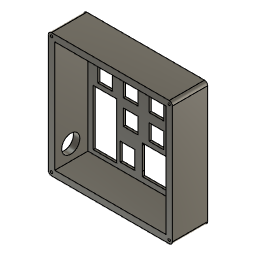
macro keyboard course ver 2 v2 (Autodesk Fusion 360 design; units mm, degrees)
Autodesk Fusion 360 part; units mm, degrees
note: some values were not read from the file. Set by a fixed rule: which sketch regions a step uses.
sketch "MacroKeyboard" plane through (0, 0, 0) normal (0, 1, 0) x (1, 0, 0)
  line L0 (24.38, -2.5067) -> (24.3899, -2.2367)
  line L1 (48.8951, -28.1499) -> (48.8951, -6.1499)
  line L2 (48.8951, -6.1499) -> (48.8951, -4.8499)
  line L3 (50.8951, -2.8499) -> (74.1951, -2.8499)
  line L4 (76.1951, -4.8499) -> (76.1951, -28.1499)
  line L5 (48.8951, -26.0859) -> (75.8951, -26.0859)
  line L6 (75.8951, -26.0859) -> (76.1951, -26.0859)
  line L7 (48.8951, -7.0859) -> (76.1951, -7.0859)
  line L8 (50.9271, -30.1499) -> (53.9271, -30.1499)
  line L9 (71.2271, -30.1499) -> (74.2271, -30.1499)
  line L10 (55.9271, -28.1499) -> (69.2271, -28.1499)
  line L11 (53.9271, -30.1499) -> (55.9271, -28.1499)
  line L12 (69.2271, -28.1499) -> (71.2271, -30.1499)
  line L13 (36.27, -14.02) -> (33.73, -14.02)
  line L14 (28.7501, -19.4501) -> (28.7501, -14.9001)
  line L15 (41.2502, -19.4501) -> (41.2502, -14.9001)
  line L16 (28.7501, -10.6) -> (28.7501, -6.05)
  line L17 (41.2502, -10.6) -> (41.2502, -6.05)
  line L18 (38.7003, -6.05) -> (41.2504, -6.05)
  line L19 (38.4002, -19.4501) -> (41.2501, -19.4501)
  line L20 (35.92, -19.4501) -> (36.62, -19.4501)
  line L21 (33.4, -19.4501) -> (34.1, -19.4501)
  line L22 (28.7501, -19.4501) -> (31.6, -19.4501)
  line L23 (33.725, -6.05) -> (36.275, -6.05)
  line L24 (28.7501, -6.05) -> (31.3, -6.05)
  line L25 (91.27, -14.02) -> (88.73, -14.02)
  line L26 (83.7501, -19.4501) -> (83.7501, -14.9001)
  line L27 (96.2502, -19.4501) -> (96.2502, -14.9001)
  line L28 (83.7501, -10.6) -> (83.7501, -6.05)
  line L29 (96.2502, -10.6) -> (96.2502, -6.05)
  line L30 (93.7003, -6.05) -> (96.2504, -6.05)
  line L31 (93.4002, -19.4501) -> (96.2501, -19.4501)
  line L32 (90.92, -19.4501) -> (91.62, -19.4501)
  line L33 (88.4, -19.4501) -> (89.1, -19.4501)
  line L34 (83.7501, -19.4501) -> (86.6, -19.4501)
  line L35 (88.725, -6.05) -> (91.275, -6.05)
  line L36 (83.7501, -6.05) -> (86.3, -6.05)
  arc A0 (48.8951, -28.1499) -> (50.8951, -30.1499) centre (50.8951, -28.1499) ccw
  arc A1 (50.8915, -2.8524) -> (48.8926, -4.8514) centre (50.8915, -4.8514) ccw
  arc A2 (76.2103, -4.8412) -> (74.2113, -2.8423) centre (74.2113, -4.8412) ccw
  arc A3 (74.1961, -30.1524) -> (76.1951, -28.1534) centre (74.1961, -28.1534) ccw
  arc A4 (36.27, -14.02) -> (33.73, -14.02) centre (35, -12.75) ccw
  arc A5 (91.27, -14.02) -> (88.73, -14.02) centre (90, -12.75) ccw
  circle A6 centre (35, -12.7501) radius 3
  circle A7 centre (90, -12.7501) radius 3
  circle A8 centre (34.1631, -39.5479) radius 0.7493
  circle A9 centre (34.1631, -39.5479) radius 1.1557
  circle A10 centre (40.5131, -37.0079) radius 0.7493
  circle A11 centre (40.5131, -37.0079) radius 1.1557
  circle A12 centre (58.2931, -39.5479) radius 0.7493
  circle A13 centre (58.2931, -39.5479) radius 1.1557
  circle A14 centre (64.6431, -37.0079) radius 0.7493
  circle A15 centre (64.6431, -37.0079) radius 1.1557
  circle A16 centre (82.4232, -39.5479) radius 0.7493
  circle A17 centre (82.4232, -39.5479) radius 1.1557
  circle A18 centre (88.7732, -37.0079) radius 0.7493
  circle A19 centre (88.7732, -37.0079) radius 1.1557
  circle A20 centre (10.287, -62.8524) radius 0.7493
  circle A21 centre (10.287, -62.8524) radius 1.1557
  circle A22 centre (16.637, -60.3124) radius 0.7493
  circle A23 centre (16.637, -60.3124) radius 1.1557
  circle A24 centre (34.163, -62.8524) radius 0.7493
  circle A25 centre (34.1631, -62.8524) radius 1.1557
  circle A26 centre (40.513, -60.3124) radius 0.7493
  circle A27 centre (40.5131, -60.3124) radius 1.1557
  circle A28 centre (58.2932, -62.8524) radius 0.7493
  circle A29 centre (58.2931, -62.8524) radius 1.1557
  circle A30 centre (64.6432, -60.3124) radius 0.7493
  circle A31 centre (64.6431, -60.3124) radius 1.1557
  circle A32 centre (82.4232, -62.8524) radius 0.7493
  circle A33 centre (82.4232, -62.8524) radius 1.1557
  circle A34 centre (88.7732, -60.3124) radius 0.7493
  circle A35 centre (88.7732, -60.3124) radius 1.1557
  circle A36 centre (10.287, -86.157) radius 0.7493
  circle A37 centre (10.287, -86.157) radius 1.1557
  circle A38 centre (16.637, -83.617) radius 0.7493
  circle A39 centre (16.637, -83.617) radius 1.1557
  circle A40 centre (34.1631, -86.157) radius 0.7493
  circle A41 centre (34.1631, -86.157) radius 1.1557
  circle A42 centre (40.5131, -83.617) radius 0.7493
  circle A43 centre (40.5131, -83.617) radius 1.1557
  circle A44 centre (58.2931, -86.157) radius 0.7493
  circle A45 centre (58.2931, -86.157) radius 1.1557
  circle A46 centre (64.6431, -83.617) radius 0.7493
  circle A47 centre (64.6431, -83.617) radius 1.1557
  circle A48 centre (82.4232, -86.157) radius 0.7493
  circle A49 centre (82.4232, -86.157) radius 1.1557
  circle A50 centre (88.7732, -83.617) radius 0.7493
  circle A51 centre (88.7732, -83.617) radius 1.1557
  arc A52 (5.0001, -4.1567) -> (5.0001, -3.0569) centre (5.0001, -3.6068) ccw
  arc A53 (4.9999, -3.0569) -> (4.9999, -4.1567) centre (4.9999, -3.6068) ccw
  line L37 (5.0001, -4.1567) -> (4.9999, -4.1567)
  line L38 (4.9999, -4.1567) -> (5.0001, -4.1567)
  line L39 (5.0001, -3.0569) -> (4.9999, -3.0569)
  line L40 (4.9999, -3.0569) -> (5.0001, -3.0569)
  arc A54 (5.0001, -6.6967) -> (5.0001, -5.5969) centre (5.0001, -6.1468) ccw
  arc A55 (4.9999, -5.5969) -> (4.9999, -6.6967) centre (4.9999, -6.1468) ccw
  line L41 (4.9999, -6.6967) -> (5.0001, -6.6967)
  line L42 (5.0001, -6.6967) -> (4.9999, -6.6967)
  line L43 (5.0001, -5.5969) -> (4.9999, -5.5969)
  line L44 (4.9999, -5.5969) -> (5.0001, -5.5969)
  arc A56 (5.0001, -9.2367) -> (5.0001, -8.1369) centre (5.0001, -8.6868) ccw
  arc A57 (4.9999, -8.1369) -> (4.9999, -9.2367) centre (4.9999, -8.6868) ccw
  line L45 (5.0001, -9.2367) -> (4.9999, -9.2367)
  line L46 (4.9999, -9.2367) -> (5.0001, -9.2367)
  line L47 (4.9999, -8.1369) -> (5.0001, -8.1369)
  line L48 (5.0001, -8.1369) -> (4.9999, -8.1369)
  arc A58 (5.0001, -11.7767) -> (5.0001, -10.6769) centre (5.0001, -11.2268) ccw
  arc A59 (4.9999, -10.6769) -> (4.9999, -11.7767) centre (4.9999, -11.2268) ccw
  line L49 (5.0001, -11.7767) -> (4.9999, -11.7767)
  line L50 (4.9999, -11.7767) -> (5.0001, -11.7767)
  line L51 (4.9999, -10.6769) -> (5.0001, -10.6769)
  line L52 (5.0001, -10.6769) -> (4.9999, -10.6769)
  arc A60 (5.0001, -14.3167) -> (5.0001, -13.2169) centre (5.0001, -13.7668) ccw
  arc A61 (4.9999, -13.2169) -> (4.9999, -14.3167) centre (4.9999, -13.7668) ccw
  line L53 (5.0001, -14.3167) -> (4.9999, -14.3167)
  line L54 (4.9999, -14.3167) -> (5.0001, -14.3167)
  line L55 (5.0001, -13.2169) -> (4.9999, -13.2169)
  line L56 (4.9999, -13.2169) -> (5.0001, -13.2169)
  arc A62 (5.0001, -16.8567) -> (5.0001, -15.7569) centre (5.0001, -16.3068) ccw
  arc A63 (4.9999, -15.7569) -> (4.9999, -16.8567) centre (4.9999, -16.3068) ccw
  line L57 (4.9999, -16.8567) -> (5.0001, -16.8567)
  line L58 (5.0001, -16.8567) -> (4.9999, -16.8567)
  line L59 (5.0001, -15.7569) -> (4.9999, -15.7569)
  line L60 (4.9999, -15.7569) -> (5.0001, -15.7569)
  arc A64 (5.0001, -19.3967) -> (5.0001, -18.2969) centre (5.0001, -18.8468) ccw
  arc A65 (4.9999, -18.2969) -> (4.9999, -19.3967) centre (4.9999, -18.8468) ccw
  line L61 (5.0001, -19.3967) -> (4.9999, -19.3967)
  line L62 (4.9999, -19.3967) -> (5.0001, -19.3967)
  line L63 (5.0001, -18.2969) -> (4.9999, -18.2969)
  line L64 (4.9999, -18.2969) -> (5.0001, -18.2969)
  arc A66 (5.0001, -21.9368) -> (5.0001, -20.8369) centre (5.0001, -21.3868) ccw
  arc A67 (4.9999, -20.8369) -> (4.9999, -21.9368) centre (4.9999, -21.3868) ccw
  line L65 (5.0001, -21.9368) -> (4.9999, -21.9368)
  line L66 (4.9999, -21.9368) -> (5.0001, -21.9368)
  line L67 (5.0001, -20.8369) -> (4.9999, -20.8369)
  line L68 (4.9999, -20.8369) -> (5.0001, -20.8369)
  arc A68 (5.0001, -24.4768) -> (5.0001, -23.3769) centre (5.0001, -23.9268) ccw
  arc A69 (4.9999, -23.3769) -> (4.9999, -24.4768) centre (4.9999, -23.9268) ccw
  line L69 (5.0001, -24.4768) -> (4.9999, -24.4768)
  line L70 (4.9999, -24.4768) -> (5.0001, -24.4768)
  line L71 (5.0001, -23.3769) -> (4.9999, -23.3769)
  line L72 (4.9999, -23.3769) -> (5.0001, -23.3769)
  arc A70 (5.0001, -27.0168) -> (5.0001, -25.9169) centre (5.0001, -26.4669) ccw
  arc A71 (4.9999, -25.9169) -> (4.9999, -27.0168) centre (4.9999, -26.4669) ccw
  line L73 (4.9999, -27.0168) -> (5.0001, -27.0168)
  line L74 (5.0001, -27.0168) -> (4.9999, -27.0168)
  line L75 (4.9999, -25.9169) -> (5.0001, -25.9169)
  line L76 (5.0001, -25.9169) -> (4.9999, -25.9169)
  arc A72 (5.0001, -29.5568) -> (5.0001, -28.4569) centre (5.0001, -29.0069) ccw
  arc A73 (4.9999, -28.4569) -> (4.9999, -29.5568) centre (4.9999, -29.0069) ccw
  line L77 (5.0001, -29.5568) -> (4.9999, -29.5568)
  line L78 (4.9999, -29.5568) -> (5.0001, -29.5568)
  line L79 (4.9999, -28.4569) -> (5.0001, -28.4569)
  line L80 (5.0001, -28.4569) -> (4.9999, -28.4569)
  arc A74 (5.0001, -32.0968) -> (5.0001, -30.997) centre (5.0001, -31.5469) ccw
  arc A75 (4.9999, -30.997) -> (4.9999, -32.0968) centre (4.9999, -31.5469) ccw
  line L81 (4.9999, -32.0968) -> (5.0001, -32.0968)
  line L82 (5.0001, -32.0968) -> (4.9999, -32.0968)
  line L83 (4.9999, -30.997) -> (5.0001, -30.997)
  line L84 (5.0001, -30.997) -> (4.9999, -30.997)
  arc A76 (5.0001, -34.6368) -> (5.0001, -33.537) centre (5.0001, -34.0869) ccw
  arc A77 (4.9999, -33.537) -> (4.9999, -34.6368) centre (4.9999, -34.0869) ccw
  line L85 (5.0001, -34.6368) -> (4.9999, -34.6368)
  line L86 (4.9999, -34.6368) -> (5.0001, -34.6368)
  line L87 (5.0001, -33.537) -> (4.9999, -33.537)
  line L88 (4.9999, -33.537) -> (5.0001, -33.537)
  arc A78 (5.0001, -37.1768) -> (5.0001, -36.077) centre (5.0001, -36.6269) ccw
  arc A79 (4.9999, -36.077) -> (4.9999, -37.1768) centre (4.9999, -36.6269) ccw
  line L89 (5.0001, -37.1768) -> (4.9999, -37.1768)
  line L90 (4.9999, -37.1768) -> (5.0001, -37.1768)
  line L91 (5.0001, -36.077) -> (4.9999, -36.077)
  line L92 (4.9999, -36.077) -> (5.0001, -36.077)
  arc A80 (5.0001, -39.7168) -> (5.0001, -38.617) centre (5.0001, -39.1669) ccw
  arc A81 (4.9999, -38.617) -> (4.9999, -39.7168) centre (4.9999, -39.1669) ccw
  line L93 (4.9999, -39.7168) -> (5.0001, -39.7168)
  line L94 (5.0001, -39.7168) -> (4.9999, -39.7168)
  line L95 (5.0001, -38.617) -> (4.9999, -38.617)
  line L96 (4.9999, -38.617) -> (5.0001, -38.617)
  arc A82 (5.0001, -42.2568) -> (5.0001, -41.157) centre (5.0001, -41.7069) ccw
  arc A83 (4.9999, -41.157) -> (4.9999, -42.2568) centre (4.9999, -41.7069) ccw
  line L97 (4.9999, -42.2568) -> (5.0001, -42.2568)
  line L98 (5.0001, -42.2568) -> (4.9999, -42.2568)
  line L99 (4.9999, -41.157) -> (5.0001, -41.157)
  line L100 (5.0001, -41.157) -> (4.9999, -41.157)
  arc A84 (5.0001, -44.7968) -> (5.0001, -43.697) centre (5.0001, -44.2469) ccw
  arc A85 (4.9999, -43.697) -> (4.9999, -44.7968) centre (4.9999, -44.2469) ccw
  line L101 (4.9999, -44.7968) -> (5.0001, -44.7968)
  line L102 (5.0001, -44.7968) -> (4.9999, -44.7968)
  line L103 (4.9999, -43.697) -> (5.0001, -43.697)
  line L104 (5.0001, -43.697) -> (4.9999, -43.697)
  arc A86 (5.0001, -47.3368) -> (5.0001, -46.237) centre (5.0001, -46.7869) ccw
  arc A87 (4.9999, -46.237) -> (4.9999, -47.3368) centre (4.9999, -46.7869) ccw
  line L105 (5.0001, -47.3368) -> (4.9999, -47.3368)
  line L106 (4.9999, -47.3368) -> (5.0001, -47.3368)
  line L107 (4.9999, -46.237) -> (5.0001, -46.237)
  line L108 (5.0001, -46.237) -> (4.9999, -46.237)
  arc A88 (5.0001, -49.8768) -> (5.0001, -48.777) centre (5.0001, -49.3269) ccw
  arc A89 (4.9999, -48.777) -> (4.9999, -49.8768) centre (4.9999, -49.3269) ccw
  line L109 (4.9999, -49.8768) -> (5.0001, -49.8768)
  line L110 (5.0001, -49.8768) -> (4.9999, -49.8768)
  line L111 (5.0001, -48.777) -> (4.9999, -48.777)
  line L112 (4.9999, -48.777) -> (5.0001, -48.777)
  arc A90 (5.0001, -52.4168) -> (5.0001, -51.317) centre (5.0001, -51.8669) ccw
  arc A91 (4.9999, -51.317) -> (4.9999, -52.4168) centre (4.9999, -51.8669) ccw
  line L113 (4.9999, -52.4168) -> (5.0001, -52.4168)
  line L114 (5.0001, -52.4168) -> (4.9999, -52.4168)
  line L115 (4.9999, -51.317) -> (5.0001, -51.317)
  line L116 (5.0001, -51.317) -> (4.9999, -51.317)
  arc A92 (22.7799, -51.317) -> (22.7799, -52.4168) centre (22.7799, -51.8669) ccw
  arc A93 (22.7802, -52.4168) -> (22.7802, -51.317) centre (22.7802, -51.8669) ccw
  line L117 (22.7799, -51.317) -> (22.7802, -51.317)
  line L118 (22.7802, -51.317) -> (22.7799, -51.317)
  line L119 (22.7799, -52.4168) -> (22.7802, -52.4168)
  line L120 (22.7802, -52.4168) -> (22.7799, -52.4168)
  arc A94 (22.7799, -48.777) -> (22.7799, -49.8768) centre (22.7799, -49.3269) ccw
  arc A95 (22.7802, -49.8768) -> (22.7802, -48.777) centre (22.7802, -49.3269) ccw
  line L121 (22.7799, -48.777) -> (22.7802, -48.777)
  line L122 (22.7802, -48.777) -> (22.7799, -48.777)
  line L123 (22.7799, -49.8768) -> (22.7802, -49.8768)
  line L124 (22.7802, -49.8768) -> (22.7799, -49.8768)
  arc A96 (22.7799, -46.237) -> (22.7799, -47.3368) centre (22.7799, -46.7869) ccw
  arc A97 (22.7802, -47.3368) -> (22.7802, -46.237) centre (22.7802, -46.7869) ccw
  line L125 (22.7802, -46.237) -> (22.7799, -46.237)
  line L126 (22.7799, -46.237) -> (22.7802, -46.237)
  line L127 (22.7802, -47.3368) -> (22.7799, -47.3368)
  line L128 (22.7799, -47.3368) -> (22.7802, -47.3368)
  arc A98 (22.7799, -43.697) -> (22.7799, -44.7968) centre (22.7799, -44.2469) ccw
  arc A99 (22.7802, -44.7968) -> (22.7802, -43.697) centre (22.7802, -44.2469) ccw
  line L129 (22.7802, -43.697) -> (22.7799, -43.697)
  line L130 (22.7799, -43.697) -> (22.7802, -43.697)
  line L131 (22.7799, -44.7968) -> (22.7802, -44.7968)
  line L132 (22.7802, -44.7968) -> (22.7799, -44.7968)
  arc A100 (22.7799, -41.157) -> (22.7799, -42.2568) centre (22.7799, -41.7069) ccw
  arc A101 (22.7802, -42.2568) -> (22.7802, -41.157) centre (22.7802, -41.7069) ccw
  line L133 (22.7799, -41.157) -> (22.7802, -41.157)
  line L134 (22.7802, -41.157) -> (22.7799, -41.157)
  line L135 (22.7802, -42.2568) -> (22.7799, -42.2568)
  line L136 (22.7799, -42.2568) -> (22.7802, -42.2568)
  arc A102 (22.7799, -38.617) -> (22.7799, -39.7168) centre (22.7799, -39.1669) ccw
  arc A103 (22.7802, -39.7168) -> (22.7802, -38.617) centre (22.7802, -39.1669) ccw
  line L137 (22.7799, -38.617) -> (22.7802, -38.617)
  line L138 (22.7802, -38.617) -> (22.7799, -38.617)
  line L139 (22.7802, -39.7168) -> (22.7799, -39.7168)
  line L140 (22.7799, -39.7168) -> (22.7802, -39.7168)
  arc A104 (22.7799, -36.077) -> (22.7799, -37.1768) centre (22.7799, -36.6269) ccw
  arc A105 (22.7802, -37.1768) -> (22.7802, -36.077) centre (22.7802, -36.6269) ccw
  line L141 (22.7802, -36.077) -> (22.7799, -36.077)
  line L142 (22.7799, -36.077) -> (22.7802, -36.077)
  line L143 (22.7802, -37.1768) -> (22.7799, -37.1768)
  line L144 (22.7799, -37.1768) -> (22.7802, -37.1768)
  arc A106 (22.7799, -33.537) -> (22.7799, -34.6368) centre (22.7799, -34.0869) ccw
  arc A107 (22.7802, -34.6368) -> (22.7802, -33.537) centre (22.7802, -34.0869) ccw
  line L145 (22.7799, -33.537) -> (22.7802, -33.537)
  line L146 (22.7802, -33.537) -> (22.7799, -33.537)
  line L147 (22.7802, -34.6368) -> (22.7799, -34.6368)
  line L148 (22.7799, -34.6368) -> (22.7802, -34.6368)
  arc A108 (22.7799, -30.997) -> (22.7799, -32.0968) centre (22.7799, -31.5469) ccw
  arc A109 (22.7802, -32.0968) -> (22.7802, -30.997) centre (22.7802, -31.5469) ccw
  line L149 (22.7802, -30.997) -> (22.7799, -30.997)
  line L150 (22.7799, -30.997) -> (22.7802, -30.997)
  line L151 (22.7802, -32.0968) -> (22.7799, -32.0968)
  line L152 (22.7799, -32.0968) -> (22.7802, -32.0968)
  arc A110 (22.7799, -28.4569) -> (22.7799, -29.5568) centre (22.7799, -29.0069) ccw
  arc A111 (22.7802, -29.5568) -> (22.7802, -28.4569) centre (22.7802, -29.0069) ccw
  line L153 (22.7802, -28.4569) -> (22.7799, -28.4569)
  line L154 (22.7799, -28.4569) -> (22.7802, -28.4569)
  line L155 (22.7799, -29.5568) -> (22.7802, -29.5568)
  line L156 (22.7802, -29.5568) -> (22.7799, -29.5568)
  arc A112 (22.7799, -25.9169) -> (22.7799, -27.0168) centre (22.7799, -26.4669) ccw
  arc A113 (22.7802, -27.0168) -> (22.7802, -25.9169) centre (22.7802, -26.4669) ccw
  line L157 (22.7802, -25.9169) -> (22.7799, -25.9169)
  line L158 (22.7799, -25.9169) -> (22.7802, -25.9169)
  line L159 (22.7799, -27.0168) -> (22.7802, -27.0168)
  line L160 (22.7802, -27.0168) -> (22.7799, -27.0168)
  arc A114 (22.7799, -23.3769) -> (22.7799, -24.4768) centre (22.7799, -23.9268) ccw
  arc A115 (22.7802, -24.4768) -> (22.7802, -23.3769) centre (22.7802, -23.9268) ccw
  line L161 (22.7799, -23.3769) -> (22.7802, -23.3769)
  line L162 (22.7802, -23.3769) -> (22.7799, -23.3769)
  line L163 (22.7799, -24.4768) -> (22.7802, -24.4768)
  line L164 (22.7802, -24.4768) -> (22.7799, -24.4768)
  arc A116 (22.7799, -20.8369) -> (22.7799, -21.9368) centre (22.7799, -21.3868) ccw
  arc A117 (22.7802, -21.9368) -> (22.7802, -20.8369) centre (22.7802, -21.3868) ccw
  line L165 (22.7802, -20.8369) -> (22.7799, -20.8369)
  line L166 (22.7799, -20.8369) -> (22.7802, -20.8369)
  line L167 (22.7799, -21.9368) -> (22.7802, -21.9368)
  line L168 (22.7802, -21.9368) -> (22.7799, -21.9368)
  arc A118 (22.7799, -18.2969) -> (22.7799, -19.3967) centre (22.7799, -18.8468) ccw
  arc A119 (22.7802, -19.3967) -> (22.7802, -18.2969) centre (22.7802, -18.8468) ccw
  line L169 (22.7799, -18.2969) -> (22.7802, -18.2969)
  line L170 (22.7802, -18.2969) -> (22.7799, -18.2969)
  line L171 (22.7802, -19.3967) -> (22.7799, -19.3967)
  line L172 (22.7799, -19.3967) -> (22.7802, -19.3967)
  arc A120 (22.7799, -15.7569) -> (22.7799, -16.8567) centre (22.7799, -16.3068) ccw
  arc A121 (22.7802, -16.8567) -> (22.7802, -15.7569) centre (22.7802, -16.3068) ccw
  line L173 (22.7799, -15.7569) -> (22.7802, -15.7569)
  line L174 (22.7802, -15.7569) -> (22.7799, -15.7569)
  line L175 (22.7802, -16.8567) -> (22.7799, -16.8567)
  line L176 (22.7799, -16.8567) -> (22.7802, -16.8567)
  arc A122 (22.7799, -13.2169) -> (22.7799, -14.3167) centre (22.7799, -13.7668) ccw
  arc A123 (22.7802, -14.3167) -> (22.7802, -13.2169) centre (22.7802, -13.7668) ccw
  line L177 (22.7802, -13.2169) -> (22.7799, -13.2169)
  line L178 (22.7799, -13.2169) -> (22.7802, -13.2169)
  line L179 (22.7802, -14.3167) -> (22.7799, -14.3167)
  line L180 (22.7799, -14.3167) -> (22.7802, -14.3167)
  arc A124 (22.7799, -10.6769) -> (22.7799, -11.7767) centre (22.7799, -11.2268) ccw
  arc A125 (22.7802, -11.7767) -> (22.7802, -10.6769) centre (22.7802, -11.2268) ccw
  line L181 (22.7802, -10.6769) -> (22.7799, -10.6769)
  line L182 (22.7799, -10.6769) -> (22.7802, -10.6769)
  line L183 (22.7799, -11.7767) -> (22.7802, -11.7767)
  line L184 (22.7802, -11.7767) -> (22.7799, -11.7767)
  arc A126 (22.7799, -8.1369) -> (22.7799, -9.2367) centre (22.7799, -8.6868) ccw
  arc A127 (22.7802, -9.2367) -> (22.7802, -8.1369) centre (22.7802, -8.6868) ccw
  line L185 (22.7799, -8.1369) -> (22.7802, -8.1369)
  line L186 (22.7802, -8.1369) -> (22.7799, -8.1369)
  line L187 (22.7799, -9.2367) -> (22.7802, -9.2367)
  line L188 (22.7802, -9.2367) -> (22.7799, -9.2367)
  arc A128 (22.7799, -5.5969) -> (22.7799, -6.6967) centre (22.7799, -6.1468) ccw
  arc A129 (22.7802, -6.6967) -> (22.7802, -5.5969) centre (22.7802, -6.1468) ccw
  line L189 (22.7799, -5.5969) -> (22.7802, -5.5969)
  line L190 (22.7802, -5.5969) -> (22.7799, -5.5969)
  line L191 (22.7802, -6.6967) -> (22.7799, -6.6967)
  line L192 (22.7799, -6.6967) -> (22.7802, -6.6967)
  arc A130 (22.7799, -3.0569) -> (22.7799, -4.1567) centre (22.7799, -3.6068) ccw
  arc A131 (22.7802, -4.1567) -> (22.7802, -3.0569) centre (22.7802, -3.6068) ccw
  line L193 (22.7802, -3.0569) -> (22.7799, -3.0569)
  line L194 (22.7799, -3.0569) -> (22.7802, -3.0569)
  line L195 (22.7802, -4.1567) -> (22.7799, -4.1567)
  line L196 (22.7799, -4.1567) -> (22.7802, -4.1567)
  arc A132 (11.8999, -51.6367) -> (10.8001, -51.6367) centre (11.35, -51.6367) ccw
  arc A133 (10.8001, -51.6369) -> (11.8999, -51.6369) centre (11.35, -51.6369) ccw
  line L197 (10.8001, -51.6369) -> (10.8001, -51.6367)
  line L198 (10.8001, -51.6367) -> (10.8001, -51.6369)
  line L199 (11.8999, -51.6367) -> (11.8999, -51.6369)
  line L200 (11.8999, -51.6369) -> (11.8999, -51.6367)
  arc A134 (14.4399, -51.6367) -> (13.3401, -51.6367) centre (13.89, -51.6367) ccw
  arc A135 (13.3401, -51.6369) -> (14.4399, -51.6369) centre (13.89, -51.6369) ccw
  line L201 (13.3401, -51.6369) -> (13.3401, -51.6367)
  line L202 (13.3401, -51.6367) -> (13.3401, -51.6369)
  line L203 (14.4399, -51.6367) -> (14.4399, -51.6369)
  line L204 (14.4399, -51.6369) -> (14.4399, -51.6367)
  arc A136 (16.9799, -51.6367) -> (15.8801, -51.6367) centre (16.43, -51.6367) ccw
  arc A137 (15.8801, -51.6369) -> (16.9799, -51.6369) centre (16.43, -51.6369) ccw
  line L205 (15.8801, -51.6367) -> (15.8801, -51.6369)
  line L206 (15.8801, -51.6369) -> (15.8801, -51.6367)
  line L207 (16.9799, -51.6367) -> (16.9799, -51.6369)
  line L208 (16.9799, -51.6369) -> (16.9799, -51.6367)
  circle A138 centre (58.8011, -4.5499) radius 0.4572
  circle A139 centre (61.3411, -4.5491) radius 0.4572
  circle A140 centre (61.3411, -4.5491) radius 0.762
  circle A141 centre (63.8811, -4.5491) radius 0.4572
  circle A142 centre (63.8811, -4.5491) radius 0.762
  circle A143 centre (66.4211, -4.5491) radius 0.4572
  circle A144 centre (66.4211, -4.5491) radius 0.762
  circle A145 centre (32.5001, -5.7501) radius 0.6
  circle A146 centre (32.5001, -5.7501) radius 0.9
  circle A147 centre (37.5001, -5.7501) radius 0.6
  circle A148 centre (37.5001, -5.7501) radius 0.9
  circle A149 centre (32.5001, -20.2499) radius 0.6
  circle A150 centre (32.5001, -20.2499) radius 0.9
  circle A151 centre (35, -20.2499) radius 0.6
  circle A152 centre (35, -20.2499) radius 0.9
  circle A153 centre (37.5001, -20.2499) radius 0.6
  circle A154 centre (37.5001, -20.2499) radius 0.9
  arc A155 (28.6, -12.0501) -> (30, -12.0501) centre (29.3, -12.0501) ccw
  arc A156 (30, -13.4501) -> (28.6, -13.4501) centre (29.3, -13.4501) ccw
  line L209 (28.6, -13.4501) -> (28.6, -12.0501)
  line L210 (28.6, -12.0501) -> (28.6, -13.4501)
  line L211 (30, -13.4501) -> (30, -12.0501)
  line L212 (30, -12.0501) -> (30, -13.4501)
  arc A157 (40, -12.0501) -> (41.4, -12.0501) centre (40.7, -12.0501) ccw
  arc A158 (41.4, -13.4501) -> (40, -13.4501) centre (40.7, -13.4501) ccw
  line L213 (40, -12.0501) -> (40, -13.4501)
  line L214 (40, -13.4501) -> (40, -12.0501)
  line L215 (41.4, -12.0501) -> (41.4, -13.4501)
  line L216 (41.4, -13.4501) -> (41.4, -12.0501)
  circle A159 centre (87.5001, -5.7501) radius 0.6
  circle A160 centre (87.5001, -5.7501) radius 0.9
  circle A161 centre (92.5001, -5.7501) radius 0.6
  circle A162 centre (92.5001, -5.7501) radius 0.9
  circle A163 centre (87.5001, -20.2499) radius 0.6
  circle A164 centre (87.5001, -20.2499) radius 0.9
  circle A165 centre (90, -20.2499) radius 0.6
  circle A166 centre (90, -20.2499) radius 0.9
  circle A167 centre (92.5001, -20.2499) radius 0.6
  circle A168 centre (92.5001, -20.2499) radius 0.9
  arc A169 (83.6, -12.0501) -> (85, -12.0501) centre (84.3, -12.0501) ccw
  arc A170 (85, -13.4501) -> (83.6, -13.4501) centre (84.3, -13.4501) ccw
  line L217 (83.6, -12.0501) -> (83.6, -13.4501)
  line L218 (83.6, -13.4501) -> (83.6, -12.0501)
  line L219 (85, -13.4501) -> (85, -12.0501)
  line L220 (85, -12.0501) -> (85, -13.4501)
  arc A171 (95, -12.0501) -> (96.4, -12.0501) centre (95.7, -12.0501) ccw
  arc A172 (96.4, -13.4501) -> (95, -13.4501) centre (95.7, -13.4501) ccw
  line L221 (95, -13.4501) -> (95, -12.0501)
  line L222 (95, -12.0501) -> (95, -13.4501)
  line L223 (96.4, -12.0501) -> (96.4, -13.4501)
  line L224 (96.4, -13.4501) -> (96.4, -12.0501)
  circle A173 centre (11.2355, -28.4567) radius 0.2
  circle A174 centre (8.2985, -33.2898) radius 0.2
  circle A175 centre (12.0828, -85.3744) radius 0.2
  circle A176 centre (90, -16.6876) radius 0.2
  circle A177 centre (43.7206, -68.8435) radius 0.2
  circle A178 centre (6.6589, -46.5507) radius 0.2
  circle A179 centre (65.2781, -49.0729) radius 0.2
  circle A180 centre (7.7234, -36.6269) radius 0.2
  circle A181 centre (37.9731, -42.0879) radius 1.9939
  circle A182 centre (62.1031, -42.0879) radius 1.9939
  circle A183 centre (86.2332, -42.0879) radius 1.9939
  circle A184 centre (14.097, -65.3924) radius 1.9939
  circle A185 centre (37.9731, -65.3924) radius 1.9939
  circle A186 centre (62.1031, -65.3924) radius 1.9939
  circle A187 centre (86.2332, -65.3924) radius 1.9939
  circle A188 centre (14.097, -88.697) radius 1.9939
  circle A189 centre (37.9731, -88.697) radius 1.9939
  circle A190 centre (62.1031, -88.697) radius 1.9939
  circle A191 centre (86.2332, -88.697) radius 1.9939
  circle A192 centre (52.1971, -28.1179) radius 1.016
  circle A193 centre (72.8981, -28.1179) radius 1.016
  circle A194 centre (52.1971, -4.9174) radius 1.016
  circle A195 centre (72.8981, -4.9174) radius 1.016
  line L225 (-2, -102) -> (-2, 2)
  line L226 (-2, 2) -> (102, 2)
  line L227 (102, 2) -> (102, -102)
  line L228 (102, -102) -> (-2, -102)
  line L229 (24.8899, -1.7367) -> (2.8899, -1.7367)
  line L230 (2.8899, -1.7367) -> (2.8899, -53.7367)
  line L231 (2.8899, -53.7367) -> (24.8899, -53.7367)
  line L232 (24.8899, -53.7367) -> (24.8899, -1.7367)
  line L233 (20.947, -96.197) -> (7.247, -96.197)
  line L234 (7.247, -96.197) -> (7.247, -81.197)
  line L235 (7.247, -81.197) -> (20.947, -81.197)
  line L236 (20.947, -81.197) -> (20.947, -96.197)
  line L237 (20.947, -96.197) -> (7.247, -81.197) construction
  line L238 (7.247, -96.197) -> (20.947, -81.197) construction
  line L239 (44.8231, -96.197) -> (31.1231, -96.197)
  line L240 (31.1231, -96.197) -> (31.1231, -81.197)
  line L241 (31.1231, -81.197) -> (44.8231, -81.197)
  line L242 (44.8231, -81.197) -> (44.8231, -96.197)
  line L243 (44.8231, -96.197) -> (31.1231, -81.197) construction
  line L244 (31.1231, -96.197) -> (44.8231, -81.197) construction
  line L245 (20.947, -72.8924) -> (7.247, -72.8924)
  line L246 (7.247, -72.8924) -> (7.247, -57.8924)
  line L247 (7.247, -57.8924) -> (20.947, -57.8924)
  line L248 (20.947, -57.8924) -> (20.947, -72.8924)
  line L249 (20.947, -72.8924) -> (7.247, -57.8924) construction
  line L250 (7.247, -72.8924) -> (20.947, -57.8924) construction
  line L251 (44.8231, -72.8924) -> (31.1231, -72.8924)
  line L252 (31.1231, -72.8924) -> (31.1231, -57.8924)
  line L253 (31.1231, -57.8924) -> (44.8231, -57.8924)
  line L254 (44.8231, -57.8924) -> (44.8231, -72.8924)
  line L255 (44.8231, -72.8924) -> (31.1231, -57.8924) construction
  line L256 (31.1231, -72.8924) -> (44.8231, -57.8924) construction
  line L257 (44.8231, -49.5879) -> (31.1231, -49.5879)
  line L258 (31.1231, -49.5879) -> (31.1231, -34.5879)
  line L259 (31.1231, -34.5879) -> (44.8231, -34.5879)
  line L260 (44.8231, -34.5879) -> (44.8231, -49.5879)
  line L261 (44.8231, -49.5879) -> (31.1231, -34.5879) construction
  line L262 (31.1231, -49.5879) -> (44.8231, -34.5879) construction
  line L263 (68.9531, -96.197) -> (55.2531, -96.197)
  line L264 (55.2531, -96.197) -> (55.2531, -81.197)
  line L265 (55.2531, -81.197) -> (68.9531, -81.197)
  line L266 (68.9531, -81.197) -> (68.9531, -96.197)
  line L267 (68.9531, -96.197) -> (55.2531, -81.197) construction
  line L268 (55.2531, -96.197) -> (68.9531, -81.197) construction
  line L269 (93.0832, -96.197) -> (79.3832, -96.197)
  line L270 (79.3832, -96.197) -> (79.3832, -81.197)
  line L271 (79.3832, -81.197) -> (93.0832, -81.197)
  line L272 (93.0832, -81.197) -> (93.0832, -96.197)
  line L273 (93.0832, -96.197) -> (79.3832, -81.197) construction
  line L274 (79.3832, -96.197) -> (93.0832, -81.197) construction
  line L275 (68.9531, -72.8924) -> (55.2531, -72.8924)
  line L276 (55.2531, -72.8924) -> (55.2531, -57.8924)
  line L277 (55.2531, -57.8924) -> (68.9531, -57.8924)
  line L278 (68.9531, -57.8924) -> (68.9531, -72.8924)
  line L279 (68.9531, -72.8924) -> (55.2531, -57.8924) construction
  line L280 (55.2531, -72.8924) -> (68.9531, -57.8924) construction
  line L281 (93.0832, -72.8924) -> (79.3832, -72.8924)
  line L282 (79.3832, -72.8924) -> (79.3832, -57.8924)
  line L283 (79.3832, -57.8924) -> (93.0832, -57.8924)
  line L284 (93.0832, -57.8924) -> (93.0832, -72.8924)
  line L285 (93.0832, -72.8924) -> (79.3832, -57.8924) construction
  line L286 (79.3832, -72.8924) -> (93.0832, -57.8924) construction
  line L287 (68.9531, -49.5879) -> (55.2531, -49.5879)
  line L288 (55.2531, -49.5879) -> (55.2531, -34.5879)
  line L289 (55.2531, -34.5879) -> (68.9531, -34.5879)
  line L290 (68.9531, -34.5879) -> (68.9531, -49.5879)
  line L291 (68.9531, -49.5879) -> (55.2531, -34.5879) construction
  line L292 (55.2531, -49.5879) -> (68.9531, -34.5879) construction
  line L293 (93.0832, -49.5879) -> (79.3832, -49.5879)
  line L294 (79.3832, -49.5879) -> (79.3832, -34.5879)
  line L295 (79.3832, -34.5879) -> (93.0832, -34.5879)
  line L296 (93.0832, -34.5879) -> (93.0832, -49.5879)
  line L297 (93.0832, -49.5879) -> (79.3832, -34.5879) construction
  line L298 (79.3832, -49.5879) -> (93.0832, -34.5879) construction
  line L299 (50.8951, -28.1499) -> (74.2113, -4.8412)
  line L300 (74.2113, -4.8412) -> (74.1961, -28.1534)
  line L301 (74.1961, -28.1534) -> (50.8915, -4.8514)
  line L302 (76.1953, -30.1524) -> (48.9111, -30.1524)
  line L303 (48.9111, -30.1524) -> (48.9111, -2.8387)
  line L304 (48.9111, -2.8387) -> (76.1953, -2.8387)
  line L305 (76.1953, -2.8387) -> (76.1953, -30.1524)
  line L306 (76.1953, -30.1524) -> (48.9111, -2.8387) construction
  line L307 (48.9111, -30.1524) -> (76.1953, -2.8387) construction
  line L308 (96.75, -21.2501) -> (83.25, -21.2501)
  line L309 (83.25, -21.2501) -> (83.25, -4.2501)
  line L310 (83.25, -4.2501) -> (96.75, -4.2501)
  line L311 (96.75, -4.2501) -> (96.75, -21.2501)
  line L312 (96.75, -21.2501) -> (83.25, -4.2501) construction
  line L313 (83.25, -21.2501) -> (96.75, -4.2501) construction
  line L314 (41.85, -21.2501) -> (28.15, -21.2501)
  line L315 (28.15, -21.2501) -> (28.15, -4.2501)
  line L316 (28.15, -4.2501) -> (41.85, -4.2501)
  line L317 (41.85, -4.2501) -> (41.85, -21.2501)
  line L318 (41.85, -21.2501) -> (28.15, -4.2501) construction
  line L319 (28.15, -21.2501) -> (41.85, -4.2501) construction
  line L320 (108, 5) -> (108, -105)
  line L321 (105, -108) -> (-5, -108)
  line L322 (-8, -105) -> (-8, 5)
  line L323 (-5, 8) -> (105, 8)
  line L324 (102, 2) -> (108, 8)
  line L325 (-8, 8) -> (-2, 2)
  line L326 (-8, -108) -> (-2, -102)
  line L327 (102, -102) -> (108, -108)
  circle A196 centre (105, -105) radius 1.1
  circle A197 centre (105, 5) radius 1.1
  circle A198 centre (-5, 5) radius 1.1
  circle A199 centre (-5, -105) radius 1.1
  arc A200 (-5, 8) -> (-8, 5) centre (-5, 5) ccw
  arc A201 (108, 5) -> (105, 8) centre (105, 5) ccw
  arc A202 (105, -108) -> (108, -105) centre (105, -105) ccw
  arc A203 (-8, -105) -> (-5, -108) centre (-5, -105) ccw
  point P0 (14.097, -88.697)
  point P1 (37.9731, -88.697)
  point P2 (14.097, -65.3924)
  point P3 (37.9731, -65.3924)
  point P4 (37.9731, -42.0879)
  point P5 (62.1031, -88.697)
  point P6 (86.2332, -88.697)
  point P7 (62.1031, -65.3924)
  point P8 (86.2332, -65.3924)
  point P9 (62.1031, -42.0879)
  point P10 (86.2332, -42.0879)
  point P11 (62.5532, -16.4956)
  point P12 (90, -12.7501)
  point P13 (35, -12.7501)
  dimension "d3" = 13.7
  dimension "d4" = 15
  dimension "d5" = 13.7
  dimension "d6" = 15
  dimension "d7" = 13.7
  dimension "d8" = 15
  dimension "d9" = 13.7
  dimension "d10" = 15
  dimension "d11" = 13.7
  dimension "d12" = 15
  dimension "d13" = 13.7
  dimension "d14" = 15
  dimension "d15" = 13.7
  dimension "d16" = 15
  dimension "d17" = 13.7
  dimension "d18" = 15
  dimension "d19" = 13.7
  dimension "d20" = 15
  dimension "d21" = 13.7
  dimension "d22" = 15
  dimension "d23" = 13.7
  dimension "d24" = 15
  dimension "d25" = 13.5
  dimension "d26" = 17
  dimension "d27" = 13.7
  dimension "d28" = 17
  dimension "d30" = 2.2
  dimension "d31" = 2.2
  dimension "d32" = 2.2
  dimension "d33" = 2.2
  dimension "d46" = 3
  dimension "d47" = 3
  dimension "d48" = 3
  dimension "d49" = 3
  constraint horizontal L233
  constraint perpendicular L233 L234
  constraint parallel L233 L235
  constraint parallel L234 L236
  constraint coincident L237 P0
  constraint coincident L238 P0
  constraint coincident P0 A188.centre
  constraint horizontal L239
  constraint perpendicular L239 L240
  constraint parallel L239 L241
  constraint parallel L240 L242
  constraint coincident L243 P1
  constraint coincident L244 P1
  constraint coincident P1 A189.centre
  constraint horizontal L245
  constraint perpendicular L245 L246
  constraint parallel L245 L247
  constraint parallel L246 L248
  constraint coincident L249 P2
  constraint coincident L250 P2
  constraint coincident P2 A184.centre
  constraint horizontal L251
  constraint perpendicular L251 L252
  constraint parallel L251 L253
  constraint parallel L252 L254
  constraint coincident L255 P3
  constraint coincident L256 P3
  constraint coincident P3 A185.centre
  constraint horizontal L257
  constraint perpendicular L257 L258
  constraint parallel L257 L259
  constraint parallel L258 L260
  constraint coincident L261 P4
  constraint coincident L262 P4
  constraint coincident P4 A181.centre
  constraint horizontal L263
  constraint perpendicular L263 L264
  constraint parallel L263 L265
  constraint parallel L264 L266
  constraint coincident L267 P5
  constraint coincident L268 P5
  constraint coincident P5 A190.centre
  constraint horizontal L269
  constraint perpendicular L269 L270
  constraint parallel L269 L271
  constraint parallel L270 L272
  constraint coincident L273 P6
  constraint coincident L274 P6
  constraint coincident P6 A191.centre
  constraint horizontal L275
  constraint perpendicular L275 L276
  constraint parallel L275 L277
  constraint parallel L276 L278
  constraint coincident L279 P7
  constraint coincident L280 P7
  constraint coincident P7 A186.centre
  constraint horizontal L281
  constraint perpendicular L281 L282
  constraint parallel L281 L283
  constraint parallel L282 L284
  constraint coincident L285 P8
  constraint coincident L286 P8
  constraint coincident P8 A187.centre
  constraint horizontal L287
  constraint perpendicular L287 L288
  constraint parallel L287 L289
  constraint parallel L288 L290
  constraint coincident L291 P9
  constraint coincident L292 P9
  constraint coincident P9 A182.centre
  constraint horizontal L293
  constraint perpendicular L293 L294
  constraint parallel L293 L295
  constraint parallel L294 L296
  constraint coincident L297 P10
  constraint coincident L298 P10
  constraint coincident P10 A183.centre
  constraint coincident A0.centre L299.start
  constraint coincident A2.centre L299.end
  constraint coincident A3.centre L300.end
  constraint coincident A1.centre L301.end
  constraint horizontal L302
  constraint perpendicular L302 L303
  constraint parallel L302 L304
  constraint parallel L303 L305
  constraint coincident L306 P11
  constraint coincident L307 P11
  constraint midpoint L299 P11
  constraint horizontal L308
  constraint perpendicular L308 L309
  constraint parallel L308 L310
  constraint parallel L309 L311
  constraint coincident L312 P12
  constraint coincident L313 P12
  constraint coincident P12 A7.centre
  constraint horizontal L314
  constraint perpendicular L314 L315
  constraint parallel L314 L316
  constraint parallel L315 L317
  constraint coincident L318 P13
  constraint coincident L319 P13
  constraint coincident P13 A6.centre
  constraint perpendicular L324 L325
  constraint perpendicular L325 L326
  constraint midpoint L327 A196.centre
  constraint midpoint L324 A197.centre
  constraint midpoint L325 A198.centre
  constraint midpoint L326 A199.centre
  constraint coincident L325.start L323
  constraint coincident L325.start L322
  constraint tangent L323 A200
  constraint tangent L322 A200
  constraint coincident L324.end L323
  constraint coincident L324.end L320
  constraint tangent L323 A201
  constraint tangent L320 A201
  constraint coincident L327.end L321
  constraint coincident L327.end L320
  constraint tangent L321 A202
  constraint tangent L320 A202
  constraint coincident L326.start L322
  constraint coincident L326.start L321
  constraint tangent L322 A203
  constraint tangent L321 A203
  measures "d3" distance of L234.end L235.end
  measures "d4" distance of L233.end L234.end
  measures "d5" distance of L240.end L241.end
  measures "d6" distance of L239.end L240.end
  measures "d7" distance of L246.end L247.end
  measures "d8" distance of L245.end L246.end
  measures "d9" distance of L252.end L253.end
  measures "d10" distance of L251.end L252.end
  measures "d11" distance of L258.end L259.end
  measures "d12" distance of L257.end L258.end
  measures "d13" distance of L264.end L265.end
  measures "d14" distance of L263.end L264.end
  measures "d15" distance of L270.end L271.end
  measures "d16" distance of L269.end L270.end
  measures "d17" distance of L276.end L277.end
  measures "d18" distance of L275.end L276.end
  measures "d19" distance of L282.end L283.end
  measures "d20" distance of L281.end L282.end
  measures "d21" distance of L288.end L289.end
  measures "d22" distance of L287.end L288.end
  measures "d23" distance of L294.end L295.end
  measures "d24" distance of L293.end L294.end
  measures "d25" distance of L309.end L310.end
  measures "d26" distance of L308.end L309.end
  measures "d27" distance of L315.end L316.end
  measures "d28" distance of L314.end L315.end
  measures "d30" diameter of A196
  measures "d31" diameter of A197
  measures "d32" diameter of A198
  measures "d33" diameter of A199 A34.centre
  measures "d46" radius of A200
  measures "d47" radius of A201
  measures "d48" radius of A202
  measures "d49" radius of A203
extrude "Extrude1" add sketch "MacroKeyboard" against normal blind 2 contours L225 L226 L227 L228
extrude "Extrude2" add sketch "MacroKeyboard" against normal blind 33 contours L225 L322 L325 L326 A198 A199 A200 A203 | L228 L321 L326 L327 A196 A199 A202 A203 | L226 L323 L324 L325 A197 A198 A200 A201 | L227 L320 L324 L327 A196 A197 A201 A202 | L326 A199 | L326 A199 | L325 A198 | L325 A198 | L327 A196 | L327 A196 | L324 A197 | L324 A197
extrude "Extrude3" cut sketch "MacroKeyboard" against normal blind 40 from surface at -20 contours L326 A199 | L326 A199 | L325 A198 | L325 A198 | L327 A196 | L327 A196 | L324 A197 | L324 A197
sketch "Sketch2" plane through (-8, 0, 0) normal (-1, 0, 0) x (0, -1, 0)
  line L0 (0, 105) -> (0, -5)
  line L1 (33, -5) -> (33, 105)
  circle A0 centre (18, 12) radius 8.5
  line L2 (0, -5) -> (33, -5)
  line L3 (33, 105) -> (0, 105)
  dimension "d41" = 17
  dimension "d43" = 18
  measures "d41" diameter of A0
  measures "d43" distance of L0 A0.centre
extrude "Extrude4" cut sketch "Sketch2" against normal blind 13 contours A0
